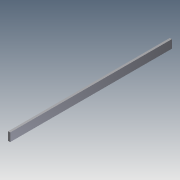
# Autodesk Inventor part: it (tech) support
Saved by Autodesk Inventor 2011 (Build 150239000, 239)
## iProperties
Created: 2011-12-03
Part Number: it (tech) support
Document SubType Name: Modeling
Designer: Matthew
Density: 1 g/cm^3
Author: Matthew
Autodesk Inventor part; units mm, degrees
ref_plane "YZ Plane" through (0, 0, 0) normal (1, 0, 0) x (0, 1, 0)
ref_plane "XZ Plane" through (0, 0, 0) normal (0, 1, 0) x (-1, 0, 0)
ref_plane "XY Plane" through (0, 0, 0) normal (0, 0, 1) x (1, 0, 0)
sketch "Sketch1" plane through (0, 0, 0) normal (0, 0, 1) x (1, 0, 0)
  line L0 (-3.0179, 9.9103) -> (3.3321, 9.9103)
  line L1 (3.3321, 9.9103) -> (3.3321, -15.4897)
  line L2 (3.3321, -15.4897) -> (-3.0179, -15.4897)
  line L3 (-3.0179, -15.4897) -> (-3.0179, 9.9103)
  point P0 (0, 0)
  dimension "d0" = 6.35
  dimension "d1" = 25.4
  constraints: 8 end point, 2 parallel, 1 horizontal, 1 perpendicular
  measures "d0" distance of L1.end L2.end
  measures "d1" distance of L0.end L1.end
extrude "Extrusion1" add sketch "Sketch1" along normal blind 495.3
body "Solid1"
